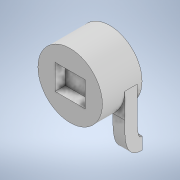
# Autodesk Inventor part: Dust Bin CFD
Saved by Autodesk Inventor 2020 (Build 240168000, 168)
## iProperties
Created: 2020-04-13
Part Number: Dust Bin CFD
Material: Generic
Document SubType Name: Modeling
Designer: pengpeng
Density: 1 g/cm^3
Appearance: Default
Author: pengpeng
Autodesk Inventor part; units mm, degrees
ref_plane "XZ Plane" through (0, 0, 0) normal (0, 1, 0) x (-1, 0, 0)
sketch "Sketch1" plane through (0, 0, 0) normal (0, 0, 1) x (1, 0, 0)
  circle A0 centre (0, 0) radius 65
  dimension "d0" = 130
  constraints: 1 centre point, 1 coincident
  measures "d0" diameter of A0
extrude "Extrusion1" add sketch "Sketch1" along normal blind 80
ref_plane "Work Plane1" through (0, 0, 35) normal (0, 0, -1) x (-1, 0, 0)
ref_plane "Work Plane2" through (65, 0, 0) normal (1, 0, 0) x (0, 1, 0)
sketch "Sketch2" plane through (0, 0, 35) normal (0, 0, -1) x (-1, 0, 0)
  circle A0 centre (0, 0) radius 65 projected
  line L0 (0, 0) -> (-65, 0) construction
  circle A1 centre (0, 0) radius 65 projected
  line L1 (-65, 0) -> (-41, 0)
  line L2 (-41, 0) -> (-41, -50.4381)
  line L3 (-41, -50.4381) -> (-65, -50.4381)
  line L4 (-65, -50.4381) -> (-65, 0)
  dimension "d4" = 24
  constraints: 10 end point, 2 horizontal, 2 parallel, 2 point on circle, 1 perpendicular, 2 other
  measures "d4" distance of L2.end L3.end
extrude "Extrusion2" add sketch "Sketch2" along normal blind 25 contours A0 L3 L4
sketch "Sketch3" plane through (65, 0, 0) normal (1, 0, 0) x (0, 1, 0)
  line L0 (0, 35) -> (-50.4381, 35) projected
  line L1 (-50.4381, 35) -> (-50.4381, 10) projected
  line L2 (0, 10) -> (-50.4381, 10) construction
  line L3 (0, 10) -> (0, 35) construction
  line L4 (0, 35) -> (-50.4381, 35) projected
  line L5 (-50.4381, 35) -> (-85.4381, 35) construction
  line L6 (-85.4381, 35) -> (-120.4381, 35) construction
  line L7 (-120.4381, 35) -> (-120.4381, 0) construction
  spline S0 degree 3 poles (-50.4381, 35) (-85.4381, 35) (-120.4381, 35) (-120.4381, 0) knots 1 1 1 1 2 2 2 2
  line L8 (0, 0) -> (-133.4667, 0) construction
  line L9 (-120.4381, 0) -> (-120.4381, 80.5106) construction
  line L10 (-50.4381, 35) -> (-166.769, 35) construction
  line L11 (111.3538, 35) -> (-213.1228, 35) construction
  dimension "d7" = 70
  dimension "d8" = 35
  dimension "d9" = 35
  constraints: 6 end point, 2 point on line, 1 collinear, 1 horizontal, 1 perpendicular, 1 vertical, 3 other
  measures "d7" distance from line of L1 L7.end
  measures "d8" distance of L7.end L6.end
  measures "d9" distance from line of L1 L5.end
sketch "Sketch4" plane through (41, -50.4381, 35) normal (0, -1, 0) x (1, 0, 0)
  line L0 (24, 0) -> (0, 0) projected
  line L1 (0, -25) -> (0, 0) projected
  line L2 (24, -25) -> (0, -25) projected
  line L3 (24, 0) -> (24, -25) projected
  point P0 (-41, -35)
sweep "Sweep1" add profiles "Sketch4" path "Sketch3" path curves S0
sketch "Sketch5" plane through (0, 0, 80) normal (0, 0, 1) x (1, 0, 0)
  circle A0 centre (0, 0) radius 65 projected
  line L0 (-30.48, 25.4) -> (30.48, 25.4)
  line L1 (30.48, 25.4) -> (30.48, -25.4)
  line L2 (30.48, -25.4) -> (-30.48, -25.4)
  line L3 (-30.48, -25.4) -> (-30.48, 25.4)
  line L4 (-30.48, 25.4) -> (30.48, -25.4) construction
  line L5 (30.48, 25.4) -> (-30.48, -25.4) construction
  dimension "d12" = 60.96
  dimension "d13" = 50.8
  constraints: 12 end point, 2 midpoint, 2 parallel, 1 horizontal, 1 perpendicular
  measures "d12" distance of L0.start L0.end
  measures "d13" distance of L0.end L1.end
extrude "Extrusion3" cut sketch "Sketch5" against normal blind 20.663 contours L0 L1 L2 L3
body "Solid1"
